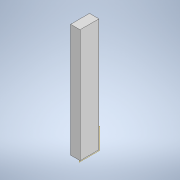
# Autodesk Inventor part: KabelBoxTest
Saved by Autodesk Inventor 2020.3 (Build 243373010, 373A)
## iProperties
Created: 2021-02-15
Part Number: KabelBoxTest
Material: Generisch
Document SubType Name: Modeling
Designer: Stefan
Density: 1 g/cm^3
Appearance: Vorgabe
Author: Stefan
Autodesk Inventor part; units mm, degrees
ref_plane "YZ Plane" through (0, 0, 0) normal (1, 0, 0) x (0, 1, 0)
ref_plane "XZ Plane" through (0, 0, 0) normal (0, 1, 0) x (-1, 0, 0)
ref_plane "XY Plane" through (0, 0, 0) normal (0, 0, 1) x (1, 0, 0)
ref_plane "Arbeitsebene1" through (16.3855, -19.5181, 0) normal (1, 0, 0) x (0, 0, -1)
sketch "Skizze2" plane through (16.3855, -19.5181, 0) normal (1, 0, 0) x (0, 0, -1)
  line L0 (0, 0) -> (-20, 0)
  line L1 (-20, 0) -> (-20, 120)
  line L2 (-20, 120) -> (0, 120)
  line L3 (0, 120) -> (0, 0)
  point P0 (0, 19.5181)
  dimension "d4" = 20
  dimension "d5" = 120
  constraints: 8 end point, 2 parallel, 1 horizontal, 1 perpendicular
  measures "d4" distance of L1.end L2.end
  measures "d5" distance of L0.end L1.end
extrude "Extrusion2" add sketch "Skizze2" along normal blind 10
